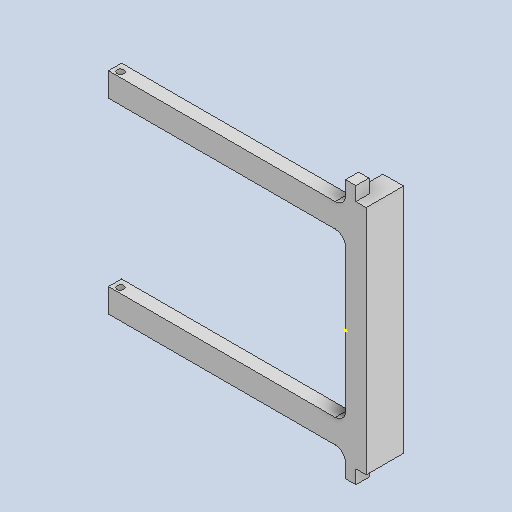
# Autodesk Inventor part: motherboard_key
Saved by Autodesk Inventor 2022 (Build 260153000, 153)
## iProperties
Created: 2024-12-17
Part Number: motherboard_key
Material: Типовые
Document SubType Name: Modeling
Designer: Andrey
Density: 1 g/cm^3
Appearance: По умолчанию
Author: Andrey
Autodesk Inventor part; units mm, degrees
ref_plane "YZ Plane" through (0, 0, 0) normal (1, 0, 0) x (0, 1, 0)
ref_plane "XZ Plane" through (0, 0, 0) normal (0, 1, 0) x (-1, 0, 0)
ref_plane "XY Plane" through (0, 0, 0) normal (0, 0, 1) x (1, 0, 0)
sketch "Эскиз8" plane through (0, 0, 0) normal (0, 0, 1) x (1, 0, 0)
  line L0 (-9, -9.9543) -> (-9, 10.0457) projected
  line L1 (0, 17.0842) -> (0, -16.9927)
  line L2 (0, 16.7842) -> (-3, 16.7842)
  line L3 (-3, 16.7842) -> (-3, -16.6927)
  line L4 (-3, -16.6927) -> (0, -16.6927)
  line L5 (0, -16.6927) -> (0, 16.7842)
  line L6 (-44, 11.5457) -> (-9, 11.5457) projected
  line L7 (-9, 15.5842) -> (-44, 15.5842) projected
  line L8 (-44, 15.5842) -> (-44, 11.5457) projected
  line L9 (-44, -15.4927) -> (-9, -15.4927) projected
  line L10 (-9, -11.4543) -> (-44, -11.4543) projected
  line L11 (-44, -11.4543) -> (-44, -15.4927) projected
  line L12 (-9, 15.2842) -> (-44, 15.2842)
  line L13 (-44, -15.1927) -> (-9, -15.1927)
  line L14 (-44, 11.8457) -> (-9.3, 11.8457)
  line L15 (-44, -11.7543) -> (-9.3, -11.7543)
  line L16 (-9.3, 15.2842) -> (-3, 15.2842)
  line L17 (-3, 15.2842) -> (-3, 11.8457)
  line L18 (-3, 11.8457) -> (-9.3, 11.8457)
  line L19 (-9.3, -11.7543) -> (-3, -11.7543)
  line L20 (-3, -11.7543) -> (-3, -15.1927)
  line L21 (-3, -15.1927) -> (-9.3, -15.1927)
  line L22 (-37.3, 15.2842) -> (-37.3, -15.1927)
  arc A0 (-10.5, -11.4543) -> (-9, -9.9543) centre (-10.5, -9.9543) ccw projected
  arc A1 (-9, 10.0457) -> (-10.5, 11.5457) centre (-10.5, 10.0457) ccw projected
  line L23 (-10.5, 11.5457) -> (-32.1754, 11.5457) projected
  line L24 (-32.1754, 11.5457) -> (-31.4296, 7.5457) projected
  line L25 (-31.4296, 7.5457) -> (-26.1754, 7.5457) projected
  line L26 (-26.1754, -4.9543) -> (-26.1754, -7.4543) projected
  line L27 (-25.1754, 4.0457) -> (-24.6192, 4.0457) projected
  line L28 (-24.6192, 4.0457) -> (-24.6192, 9.5457) projected
  spline S0 degree 3 poles (-24.1006, 10.0457) (-24.1642, 10.0457) (-24.2391, 10.0312) (-24.3567, 9.984) (-24.4205, 9.943) (-24.5115, 9.8556) (-24.5549, 9.7937) (-24.6042, 9.6794) (-24.6192, 9.6072) (-24.6192, 9.5457) knots 0.074888 0.074888 0.074888 0.074888 0.093967 0.093967 0.112918 0.112918 0.131824 0.131824 0.15026 0.15026 0.15026 0.15026 projected
  line L29 (-24.1006, 10.0457) -> (-24.0379, 10.0457) projected
  spline S1 degree 3 poles (-23.5192, 9.5457) (-23.5192, 9.6072) (-23.5343, 9.6794) (-23.5836, 9.7937) (-23.6269, 9.8556) (-23.718, 9.943) (-23.7817, 9.984) (-23.8994, 10.0312) (-23.9743, 10.0457) (-24.0379, 10.0457) knots 0.15026 0.15026 0.15026 0.15026 0.168696 0.168696 0.187602 0.187602 0.206553 0.206553 0.225632 0.225632 0.225632 0.225632 projected
  line L30 (-23.5192, 9.5457) -> (-23.5192, 4.0457) projected
  line L31 (-22.8192, 4.0457) -> (-22.8192, -3.9543) projected
  line L32 (-22.8192, -3.9543) -> (-23.5192, -3.9543) projected
  line L33 (-23.5192, -3.9543) -> (-23.5192, -9.4543) projected
  spline S2 degree 3 poles (-24.0379, -9.9543) (-23.9743, -9.9543) (-23.8994, -9.9398) (-23.7817, -9.8925) (-23.718, -9.8516) (-23.6269, -9.7642) (-23.5836, -9.7022) (-23.5343, -9.5879) (-23.5192, -9.5157) (-23.5192, -9.4543) knots 0.074888 0.074888 0.074888 0.074888 0.093967 0.093967 0.112918 0.112918 0.131824 0.131824 0.15026 0.15026 0.15026 0.15026 projected
  line L34 (-24.0379, -9.9543) -> (-24.1006, -9.9543) projected
  spline S3 degree 3 poles (-24.6192, -9.4543) (-24.6192, -9.5157) (-24.6042, -9.5879) (-24.5549, -9.7022) (-24.5115, -9.7642) (-24.4205, -9.8516) (-24.3567, -9.8925) (-24.2391, -9.9398) (-24.1642, -9.9543) (-24.1006, -9.9543) knots 0.15026 0.15026 0.15026 0.15026 0.168696 0.168696 0.187602 0.187602 0.206553 0.206553 0.225632 0.225632 0.225632 0.225632 projected
  line L35 (-24.6192, -9.4543) -> (-24.6192, -3.9543) projected
  line L36 (-24.6192, -3.9543) -> (-25.1754, -3.9543) projected
  line L37 (-26.1754, 7.5457) -> (-26.1754, 5.0457) projected
  line L38 (-26.1754, -7.4543) -> (-31.4296, -7.4543) projected
  line L39 (-31.4296, -7.4543) -> (-32.1754, -11.4543) projected
  line L40 (-32.1754, -11.4543) -> (-10.5, -11.4543) projected
  line L41 (-26.1754, -4.9543) -> (-25.1754, -3.9543) projected
  line L42 (-25.1754, 4.0457) -> (-26.1754, 5.0457) projected
  line L43 (-23.5192, 4.0457) -> (-22.8192, 4.0457) projected
  point P0 (0, 0)
  point P1 (-32.1754, 15.5842)
  point P2 (-32.1754, -15.4927)
  point P3 (0, -16.6927)
  point P4 (-3, 15.2842)
  point P5 (-37.3, 11.8457)
  point P6 (-9.3, 11.8457)
  point P7 (-37.3, -11.7543)
  point P8 (-9, -15.1927)
  dimension "d40" = 3
  dimension "d43" = 0.3
  dimension "d44" = 0.3
  dimension "d45" = 0.3
  dimension "d46" = 0.3
  dimension "d47" = 6.7
  constraints: 32 end point, 6 parallel, 6 point on line, 4 perpendicular, 3 horizontal, 2 collinear, 1 vertical
  measures "d40" distance of L4.end L3.end
  measures "d43" distance between parallel lines of L7 L12
  measures "d44" distance between parallel lines of L9 L13
  measures "d45" distance between parallel lines of L6 L14
  measures "d46" distance between parallel lines of L10 L15
  measures "d47" distance from line of L14.start L22
extrude "Выдавливание8" add sketch "Эскиз8" against normal blind 1.9 contours L15 L19 L3 L21 L13 L22 | L22 L12 L16 L3 L18 L14 | L3 L2 L1 L4
sketch "Эскиз9" plane through (0, 0, -1.9) normal (0, 0, -1) x (-1, 0, 0)
  line L0 (0, 16.7842) -> (0, -16.6927) projected
  line L1 (0, -16.6927) -> (3, -16.6927) projected
  line L2 (3, -16.6927) -> (3, -15.1927) projected
  line L3 (3, -15.1927) -> (37.3, -15.1927) projected
  line L4 (37.3, -15.1927) -> (37.3, -11.7543) projected
  line L5 (37.3, -11.7543) -> (3, -11.7543) projected
  line L6 (3, -11.7543) -> (3, 11.8457) projected
  line L7 (3, 11.8457) -> (37.3, 11.8457) projected
  line L8 (37.3, 11.8457) -> (37.3, 15.2842) projected
  line L9 (37.3, 15.2842) -> (3, 15.2842) projected
  line L10 (3, 15.2842) -> (3, 16.7842) projected
  line L11 (3, 16.7842) -> (0, 16.7842) projected
  line L12 (37.3, 15.2842) -> (3, 15.2842) projected
  line L13 (3, -15.1927) -> (37.3, -15.1927) projected
  line L14 (3, 15.2842) -> (3, -15.1927)
  point P0 (0, 0)
  point P1 (3, -11.7543)
  constraints: 2 end point, 1 perpendicular
extrude "Выдавливание9" add sketch "Эскиз9" along normal blind 3.5 contours L11 L10 L14 L6 L2 L1 L0
fillet "Сопряжение9" radius 1.5 4 edges at (-3, 15.2842, -0.95) (-3, 11.8457, -0.95) (-3, -11.7543, -0.95) (-3, -15.1927, -0.95)
sketch "Эскиз10" plane through (-3, -16.6927, -5.4) normal (-1, 0, 0) x (0, 0, 1)
  arc A0 (1.4727, 14.8527) -> (1.4727, 18.6243) centre (2.7, 16.7385) ccw projected
  circle A1 centre (2.7, 16.7385) radius 2.25
  point P0 (5.4, 16.6927)
  point P1 (1.4727, 18.6243)
  constraints: 1 coincident, 3 other
extrude "Выдавливание10" cut sketch "Эскиз10" against normal blind 1.5
sketch "Эскиз11" plane through (-3, -16.6927, -5.4) normal (-1, 0, 0) x (0, 0, 1)
  point P0 (5.4, 16.6927)
sketch "Эскиз12" plane through (-3, -16.6927, -5.4) normal (-1, 0, 0) x (0, 0, 1)
  circle A0 centre (2.7, 16.7385) radius 2.25 projected
  line L0 (3.5, 6.4385) -> (3.5, 0) projected
  line L1 (5.4, 6.4385) -> (3.5, 6.4385) projected
  line L2 (5.4, 27.0385) -> (5.4, 6.4385) projected
  line L3 (3.5, 27.0385) -> (5.4, 27.0385) projected
  line L4 (3.5, 33.4769) -> (3.5, 27.0385) projected
  line L5 (3.5, 33.4769) -> (0, 33.4769) projected
  line L6 (0, 0) -> (0, 33.4769) projected
  line L7 (3.5, 0) -> (0, 0) projected
  line L8 (3.5, 1.5) -> (3.5, 0) projected
  line L9 (5.4, 0) -> (3.5, 0) projected
  line L10 (5.4, 0) -> (5.4, 1.5) projected
  line L11 (5.4, 1.5) -> (3.5, 1.5) projected
  line L12 (5.4, 33.4769) -> (0, 33.4769) projected
  line L13 (5.4, 0) -> (3.5, 0)
  line L14 (3.5, 0) -> (3.5, -2)
  line L15 (3.5, -2) -> (5.4, -2)
  line L16 (5.4, -2) -> (5.4, 0)
  line L17 (3.5, 6.4385) -> (3.5, 0) projected
  line L18 (5.4, 33.4769) -> (3.5, 33.4769) projected
  line L19 (5.4, 33.4769) -> (3.5, 33.4769)
  line L20 (3.5, 33.4769) -> (3.5, 35.4769)
  line L21 (3.5, 35.4769) -> (5.4, 35.4769)
  line L22 (5.4, 35.4769) -> (5.4, 33.4769)
  line L23 (3.5, 33.4769) -> (3.5, 27.0385) projected
  point P0 (5.4, 16.6927)
  dimension "d56" = 2
  dimension "d57" = 2
  constraints: 16 end point, 4 parallel, 2 collinear, 2 horizontal, 2 perpendicular
  measures "d56" distance of L14.end L13.end
  measures "d57" distance of L19.end L20.end
extrude "Выдавливание11" add sketch "Эскиз12" against normal blind 1.5 contours L20 L21 L22 L12 | L9 L16 L15 L14
sketch "Эскиз13" plane through (-37.3, 15.2842, 0) normal (0, 1, 0) x (1, 0, 0)
  line L0 (32.8, 1.9) -> (32.8, 0) projected
  line L1 (0, 1.9) -> (32.8, 1.9) projected
  line L2 (0, 0) -> (0, 1.9) projected
  line L3 (32.8, 0) -> (0, 0) projected
  circle A0 centre (1, 0.75) radius 0.5
  circle A1 centre (1, 0.75) radius 0.75
  line L4 (1, 0.75) -> (0, 0.75)
  point P0 (37.3, 0)
  dimension "d60" = 1
  dimension "d61" = 1.5
  dimension "d62" = 1
  constraints: 2 centre point, 2 end point, 1 coincident, 1 parallel, 1 point on line, 1 tangent
  measures "d60" diameter of A0
  measures "d61" diameter of A1
  measures "d62" distance of L4.start L4.end
extrude "Выдавливание12" cut sketch "Эскиз13" against normal blind 40 contours A0
